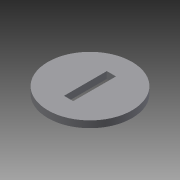
# Autodesk Inventor part: open2
Saved by Autodesk Inventor 2015 (Build 190159000, 159)
## iProperties
Created: 2015-02-17
Part Number: open2
Material: Generic
Document SubType Name: Modeling
Designer: Hanjie
Density: 1 g/cm^3
Appearance: Default
Author: Hanjie
Autodesk Inventor part; units mm, degrees
ref_plane "YZ Plane" through (0, 0, 0) normal (1, 0, 0) x (0, 1, 0)
ref_plane "XZ Plane" through (0, 0, 0) normal (0, 1, 0) x (-1, 0, 0)
ref_plane "XY Plane" through (0, 0, 0) normal (0, 0, 1) x (1, 0, 0)
sketch "Sketch1" plane through (0, 0, 0) normal (0, 1, 0) x (-1, 0, 0)
  circle A0 centre (0, 0) radius 34.925
  dimension "d0" = 69.85
  constraints: 1 centre point, 1 coincident
  measures "d0" diameter of A0
extrude "Extrusion1" add sketch "Sketch1" along normal blind 5.588
sketch "Sketch2" plane through (0, 5.588, 0) normal (0, 1, 0) x (1, 0, 0)
  line L0 (0, 0) -> (0, -17.78)
  line L1 (0, -17.78) -> (-3.81, -17.78)
  line L2 (-3.81, -17.78) -> (3.81, -17.78)
  line L3 (3.81, -17.78) -> (3.81, 17.78)
  line L4 (3.81, 17.78) -> (-3.81, 17.78)
  line L5 (-3.81, 17.78) -> (-3.81, -17.78)
  dimension "d3" = 17.78
  dimension "d4" = 3.81
  dimension "d5" = 7.62
  dimension "d6" = 35.56
  constraints: 12 end point, 2 parallel, 2 perpendicular, 1 horizontal, 1 vertical
  measures "d3" distance of L0.start L0.end
  measures "d4" distance of L0.end L1.end
  measures "d5" distance of L4.end L3.end
  measures "d6" distance of L3.end L2.end
extrude "Extrusion2" cut sketch "Sketch2" against normal blind 5.588
body "Solid1"
